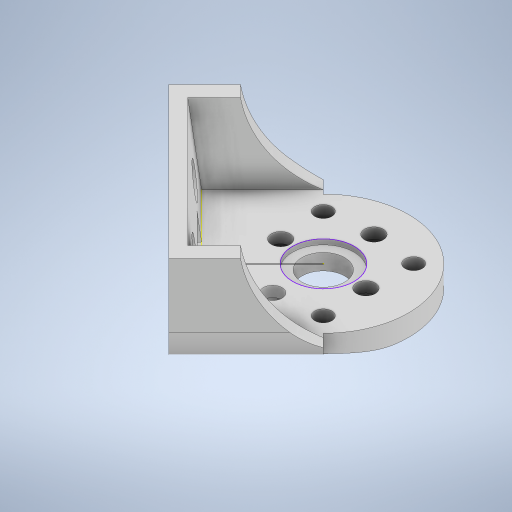
# Autodesk Inventor part: SoporteV4
Saved by Autodesk Inventor 2024 (Build 280153000, 153)
## iProperties
Created: 2023-09-30
Part Number: SoporteV4
Material: Generic
Document SubType Name: Modeling
Designer: felip
Density: 1 g/cm^3
Appearance: Default
Author: felip
Autodesk Inventor part; units mm, degrees
ref_plane "YZ Plane" through (0, 0, 0) normal (1, 0, 0) x (0, 1, 0)
ref_plane "XZ Plane" through (0, 0, 0) normal (0, 1, 0) x (-1, 0, 0)
sketch "Sketch1" plane through (0, 0, 0) normal (0, 1, 0) x (-1, 0, 0)
  line L0 (0, 0) -> (8, 0)
  line L1 (0, 0) -> (-8, 0)
  line L2 (0, 0) -> (0, -9.5)
  line L3 (0, -9.5) -> (0, 9.5)
  circle A0 centre (0, 0) radius 16
  circle A1 centre (0, 9.5) radius 1.75
  circle A2 centre (8, 0) radius 1.75
  circle A3 centre (0, -9.5) radius 1.75
  circle A4 centre (-8, 0) radius 1.75
  circle A5 centre (0, 0) radius 4
  circle A6 centre (0, -9.5) radius 3
  circle A7 centre (8, 0) radius 3
  circle A8 centre (0, 9.5) radius 3
  circle A9 centre (-8, 0) radius 3
  point P0 (16, 0)
  point P1 (0, 16)
  dimension "d0" = 8
  dimension "d1" = 8
  dimension "d2" = 9.5
  dimension "d3" = 19
  dimension "d4" = 32
  dimension "d5" = 3.5
  dimension "d6" = 3.5
  dimension "d7" = 3.5
  dimension "d8" = 3.5
  dimension "d9" = 8
  dimension "d10" = 6
  dimension "d11" = 6
  dimension "d12" = 6
  dimension "d13" = 6
  constraints: 10 centre point, 10 coincident, 8 end point, 2 horizontal, 2 point on circle, 1 point on line, 1 vertical
  measures "d0" distance of L0.start L0.end
  measures "d1" distance of L0.start L1.end
  measures "d2" distance of L0.start L2.end
  measures "d3" distance of L2.end L3.end
  measures "d4" diameter of A0
  measures "d5" diameter of A1
  measures "d6" diameter of A2
  measures "d7" diameter of A3
  measures "d8" diameter of A4
  measures "d9" diameter of A5
  measures "d10" diameter of A6
  measures "d11" diameter of A7
  measures "d12" diameter of A8
  measures "d13" diameter of A9
extrude "Extrusion1" add sketch "Sketch1" along normal blind 4 contours A0
sketch "Sketch3" plane through (0, 4, 0) normal (0, 1, 0) x (1, 0, 0)
  circle A0 centre (0, -9.5) radius 3 projected
  circle A1 centre (0, -9.5) radius 1.75
  circle A2 centre (-8, 0) radius 3 projected
  circle A3 centre (-8, 0) radius 1.75
  circle A4 centre (0, 9.5) radius 3 projected
  circle A5 centre (0, 9.5) radius 1.75
  circle A6 centre (8, 0) radius 3 projected
  circle A7 centre (8, 0) radius 1.75
  point P0 (0, 0)
  dimension "d16" = 3.5
  dimension "d17" = 3.5
  dimension "d18" = 3.5
  dimension "d19" = 3.5
  constraints: 4 centre point, 4 coincident
  measures "d16" diameter of A1
  measures "d17" diameter of A3
  measures "d18" diameter of A5
  measures "d19" diameter of A7
extrude "Extrusion2" add sketch "Sketch3" against normal blind 2
sketch "Sketch5" plane through (0, 0, 0) normal (0, -1, 0) x (1, 0, 0)
  line L0 (0, 0) -> (-4, 0)
  circle A0 centre (0, 0) radius 4 projected
  line L1 (0, 0) -> (0, 4)
  line L2 (0, 0) -> (-14.8492, 14.8492)
  line L3 (0, 0) -> (21, 0) construction
  line L4 (-14.8492, 14.8492) -> (-21.9203, 7.7782)
  line L5 (-14.8492, 14.8492) -> (-7.7782, 21.9203)
  line L6 (-21.9203, 7.7782) -> (-15.683, 1.5408)
  line L7 (-7.7782, 21.9203) -> (-0.7071, 14.8492)
  line L8 (-0.7071, 14.8492) -> (-15.683, 1.5408)
  point P0 (-8.195, 8.195)
  point P1 (-2.8284, 2.8284)
  dimension "d22" = 21
  dimension "d23" = 135
  dimension "d24" = 10
  dimension "d28" = 10
  constraints: 18 end point, 2 horizontal, 2 point on circle, 1 equal length, 1 vertical
  measures "d22" distance of L1.start L2.end
  measures "d23" angle of L3 L2
  measures "d24" distance of L2.end L4.end
  measures "d28" distance of L2.end L5.end
extrude "Extrusion3" add sketch "Sketch5" against normal blind 5 contours L8 L6 L4 L2 | L2 L5 L7 L8
sketch "Sketch6" plane through (0, 0, 0) normal (0, -1, 0) x (1, 0, 0)
  line L0 (-21.9203, 7.7782) -> (-7.7782, 21.9203) projected
  line L1 (-7.7782, 21.9203) -> (-21.9203, 7.7782)
  line L2 (-21.9203, 7.7782) -> (-19.799, 5.6569)
  line L3 (-19.799, 5.6569) -> (-5.6569, 19.799)
  line L4 (-5.6569, 19.799) -> (-7.7782, 21.9203)
  point P0 (0, 0)
  dimension "d31" = 20
  dimension "d32" = 3
  constraints: 8 end point, 2 parallel, 1 perpendicular, 1 point on line
  measures "d31" distance of L0.end L1.end
  measures "d32" distance of L2.end L1.end
extrude "Extrusion4" add sketch "Sketch6" along normal blind 17
sketch "Sketch7" plane through (0, 0, 0) normal (0, -1, 0) x (1, 0, 0)
  circle A0 centre (0, 0) radius 4 projected
  line L0 (0, 0) -> (-10.6066, 10.6066)
  line L1 (0, 0) -> (15, 0) construction
  dimension "d36" = 15
  dimension "d37" = 135
  constraints: 4 end point, 1 equal length, 1 horizontal
  measures "d36" distance of L0.start L0.end
  measures "d37" angle of L1 L0
sketch "Sketch8" plane through (-5.6569, -17, 19.799) normal (0.7071068, 0, -0.7071068) x (-0.7071068, 0, -0.7071068)
  line L0 (10, 17) -> (10, 0)
  line L1 (20, 0) -> (0, 0) projected
  constraints: 2 end point, 1 midpoint
ref_plane "Work Plane3" through (0, 0, 0) normal (0.7071068, 0, 0.7071068) x (-0.7071068, 0, 0.7071068)
sketch "Sketch11" plane through (-5.6569, -17, 19.799) normal (0.7071068, 0, -0.7071068) x (-0.7071068, 0, -0.7071068)
  line L0 (0, 17) -> (20, 17) projected
  line L1 (20, 22) -> (20, 0) projected
  line L2 (0, 17) -> (20, 17)
  line L3 (20, 17) -> (20, 2)
  line L4 (20, 2) -> (0, 2)
  line L5 (0, 2) -> (0, 17)
  line L6 (0, 17) -> (4, 17)
  line L7 (4, 17) -> (4, 14)
  line L8 (4, 14) -> (4, 6)
  line L9 (4, 6) -> (16, 6)
  line L10 (16, 6) -> (16, 14)
  circle A0 centre (4, 14) radius 1.75
  circle A1 centre (4, 6) radius 1.75
  circle A2 centre (16, 6) radius 1.75
  circle A3 centre (16, 14) radius 1.75
  point P0 (10, 17)
  point P1 (8.5, 15)
  dimension "d48" = 4
  dimension "d49" = 3
  dimension "d50" = 8
  dimension "d51" = 12
  dimension "d52" = 8
  dimension "d53" = 3.5
  dimension "d54" = 3.5
  dimension "d55" = 3.5
  dimension "d56" = 3.5
  constraints: 18 end point, 4 centre point, 4 coincident, 3 perpendicular, 2 horizontal, 2 parallel, 2 point on line, 1 vertical, 1 other
  measures "d48" distance of L2.start L6.end
  measures "d49" distance of L6.end L7.end
  measures "d50" distance of L7.end L8.end
  measures "d51" distance of L8.end L9.end
  measures "d52" distance of L9.end L10.end
  measures "d53" diameter of A0
  measures "d54" diameter of A1
  measures "d55" diameter of A2
  measures "d56" diameter of A3
extrude "Extrusion7" cut sketch "Sketch11" against normal blind 5 contours A0 L8 L7 | L7 L8 A0 | A1 L9 L8 | L8 L9 A1 | A2 L10 L9 | L9 L10 A2 | A3
sketch "Sketch12" plane through (0, 0, 0) normal (0, -1, 0) x (1, 0, 0)
  line L0 (0, 0) -> (-8.4853, -8.4853)
  line L1 (0, 0) -> (12, 0) construction
  circle A0 centre (-8.4853, -8.4853) radius 1.6
  line L2 (0, 0) -> (8.4853, -8.4853)
  circle A1 centre (8.4853, -8.4853) radius 1.6
  line L3 (0, 0) -> (8.4853, 8.4853)
  circle A2 centre (8.4853, 8.4853) radius 1.6
  line L4 (0, 0) -> (-8.4853, 8.4853)
  circle A3 centre (-8.4853, 8.4853) radius 1.6
  line L5 (0, 0) -> (-11.5258, 11.5258)
  line L6 (0, 0) -> (11.5258, 11.5258)
  line L7 (11.5258, 11.5258) -> (-11.5258, 11.5258)
  dimension "d60" = 12
  dimension "d61" = 135
  dimension "d62" = 3.2
  dimension "d63" = 12
  dimension "d64" = 3.2
  dimension "d65" = 12
  dimension "d66" = 3.2
  dimension "d69" = 12
  dimension "d70" = 3.2
  dimension "d71" = 16.3
  dimension "d75" = 16.3
  constraints: 16 end point, 4 centre point, 4 coincident, 2 horizontal, 2 point on line, 1 equal length
  measures "d60" distance of L0.start L0.end
  measures "d61" angle of L0 L1
  measures "d62" diameter of A0
  measures "d63" distance of L0.start L2.end
  measures "d64" diameter of A1
  measures "d65" distance of L3.start L3.end
  measures "d66" diameter of A2
  measures "d69" distance of L3.start L4.end
  measures "d70" diameter of A3
  measures "d71" distance of L3.start L5.end
  measures "d75" distance of L3.start L6.end
sketch "Sketch13" plane through (0, 4, 0) normal (0, 1, 0) x (1, 0, 0)
  circle A0 centre (0, 0) radius 5.75
  dimension "d72" = 11.5
  constraints: 1 centre point, 1 coincident
  measures "d72" diameter of A0
extrude "Extrusion8" cut sketch "Sketch13" against normal blind 1
sketch "Sketch14" plane through (-1.7398, 0, 15.882) normal (0.7071068, 0, 0.7071068) x (0.7071068, 0, -0.7071068)
  line L0 (-8.5395, 5) -> (-8.5395, -17) projected
  line L1 (-8.5395, -17) -> (-8.5395, 5)
  line L2 (-8.5395, 5) -> (6.4605, 5)
  line L3 (3.6299, 5) -> (-0.0177, 5) projected
  line L4 (6.4605, 5) -> (-8.5395, -17)
  point P0 (12.4605, 0)
  dimension "d76" = 15
  constraints: 6 end point, 1 collinear, 1 point on line
  measures "d76" distance of L0.start L2.end
extrude "Extrusion9" add sketch "Sketch14" along normal blind 3
fillet "Fillet3" radius 1 3 edges at (-5.6569, -14.8, 19.799) (-6.7175, -17, 20.8597) (-1.53, -8.4401, 19.9147)
sketch "Sketch15" plane through (-15.683, 0, 1.5408) normal (-0.7071068, 0, -0.7071068) x (-0.7071068, 0, 0.7071068)
  line L0 (8.821, 5) -> (8.821, -17) projected
  line L1 (8.821, -17) -> (8.821, 5)
  line L2 (8.821, 5) -> (-6.179, 5)
  line L3 (-6.179, 5) -> (8.821, -17)
  point P0 (-12.179, 0)
  dimension "d80" = 15
  constraints: 6 end point, 1 perpendicular, 1 vertical
  measures "d80" distance of L0.start L2.end
extrude "Extrusion10" add sketch "Sketch15" along normal blind 3
fillet "Fillet4" radius 1 3 edges at (-19.799, -14.8, 5.6569) (-20.8597, -17, 6.7175) (-19.9147, -8.4401, 1.53)
extrude "Extrusion11" cut sketch "Sketch12" against normal blind 6 contours A0 | A1 | A2 L6 L3 | L3 L6 A2 | A3 L5 L4 | L4 L5 A3
sketch "Sketch16" plane through (0, 5, 0) normal (0, 1, 0) x (1, 0, 0)
  line L0 (-5.6569, -24.0416) -> (-24.0416, -5.6569) projected
  line L1 (-24.0416, -5.6569) -> (-13.3457, 5.0391)
  line L2 (-13.3457, 5.0391) -> (5.0391, -13.3457)
  line L3 (5.0391, -13.3457) -> (-5.6569, -24.0416)
  line L4 (-5.6569, -24.0416) -> (-24.0416, -5.6569)
  point P0 (0, 0)
  point P1 (-5.6569, -24.0416)
  constraints: 8 end point, 2 parallel, 2 perpendicular
extrude "Extrusion12" cut sketch "Sketch16" against normal blind 1
sketch "Sketch17" plane through (0, 4, 0) normal (0, 1, 0) x (1, 0, 0)
  line L0 (-17.21, -2.4586) -> (-13.6377, 2.2484)
  line L1 (-13.6377, 2.2484) -> (-11.5469, 0.6617)
  line L2 (-11.5469, 0.6617) -> (-15.1192, -4.0453)
  line L3 (-15.1192, -4.0453) -> (-17.21, -2.4586)
  point P0 (0, 0)
  constraints: 8 end point, 2 parallel, 1 perpendicular
extrude "Extrusion13" add sketch "Sketch17" against normal blind 4
sketch "Sketch18" plane through (-5.6569, -12.6, 19.799) normal (0.7071068, 0, -0.7071068) x (-0.7071068, 0, -0.7071068)
  line L0 (10, 12.6) -> (10, -4.4)
  line L1 (19, -4.4) -> (1, -4.4) projected
  line L2 (10, 12.6) -> (10, 4.1)
  line L3 (10, 4.1) -> (24.9533, 4.1)
  line L4 (24.9533, 4.1) -> (-2.995, 4.1)
  line L5 (24.9533, 4.1) -> (-3.5693, 4.1)
  line L6 (-3.5693, 4.1) -> (-3.5693, -4.8148)
  line L7 (-3.5693, -4.8148) -> (24.9533, -4.8148)
  line L8 (24.9533, -4.8148) -> (24.9533, 4.1)
  point P0 (10, 4.1)
  dimension "d90" = 8.5
  constraints: 16 end point, 2 midpoint, 2 parallel, 2 perpendicular, 1 horizontal, 1 point on line
  measures "d90" distance of L0.start L2.end
extrude "Extrusion14" cut sketch "Sketch18" along normal mid plane 10
fillet "Fillet5" radius 2 1 edges at (-12.7279, -8.5, 12.7279)
sketch "Sketch19" plane through (0, 0, 0) normal (0, -1, 0) x (1, 0, 0)
  line L0 (0, 0) -> (12.0208, 12.0208)
  line L1 (0, 0) -> (17, 0) construction
  line L2 (0, 0) -> (-12.0208, -12.0208)
  line L3 (0, 0) -> (-14.8492, 14.8492)
  line L4 (-5.6569, 24.0416) -> (-24.0416, 5.6569) projected
  line L5 (-14.8492, 14.8492) -> (-26.8701, 2.8284)
  line L6 (-26.8701, 2.8284) -> (-12.0208, -12.0208)
  line L7 (-14.8492, 14.8492) -> (-2.8284, 26.8701)
  line L8 (-2.8284, 26.8701) -> (12.0208, 12.0208)
  arc A0 (-15.8638, -2.0835) -> (2.0835, 15.8638) centre (0, 0) ccw projected
  line L9 (-23.8901, 5.8084) -> (-13.0815, -5.0003)
  line L10 (-13.0815, -5.0003) -> (-11.3137, -11.3137)
  line L11 (-6.0104, 23.6881) -> (6.62, 11.0576)
  line L12 (6.62, 11.0576) -> (11.3137, 11.3137)
  point P0 (-15.8425, -2.2392)
  point P1 (-24.0416, 5.6569)
  dimension "d96" = 17
  dimension "d97" = 45
  dimension "d98" = 17
  dimension "d99" = 17
  dimension "d100" = 17
  constraints: 24 end point, 6 point on line, 3 perpendicular, 2 point on circle, 1 equal length, 1 horizontal, 1 midpoint
  measures "d96" distance of L0.start L0.end
  measures "d97" angle of L1 L0
  measures "d98" distance of L0.start L2.end
  measures "d99" distance of L3.end L5.end
  measures "d100" distance of L3.end L7.end
extrude "Extrusion15" add sketch "Sketch19" against normal blind 4 contours L12 L11 L4 L7 L8 L0 | L2 L6 L5 L4 L9 A0
sketch "Sketch21" plane through (0, 0, 0) normal (0, -1, 0) x (1, 0, 0)
  line L0 (12.0208, 12.0208) -> (-2.8284, 26.8701) projected
  line L1 (12.0208, 12.0208) -> (14.1421, 14.1421)
  line L2 (12.0208, 12.0208) -> (15.0208, 12.0208) construction
  line L3 (14.1421, 14.1421) -> (-0.7071, 28.9914)
  line L4 (-0.7071, 28.9914) -> (-2.8284, 26.8701)
  line L5 (-2.8284, 26.8701) -> (-5.6569, 24.0416) projected
  line L6 (-2.8284, 26.8701) -> (12.0208, 12.0208)
  line L7 (-11.3137, -11.3137) -> (-12.0208, -12.0208) projected
  line L8 (-12.0208, -12.0208) -> (-14.1421, -14.1421)
  line L9 (-14.1421, -14.1421) -> (-28.9914, 0.7071)
  line L10 (-26.8701, 2.8284) -> (-12.0208, -12.0208) projected
  line L11 (-28.9914, 0.7071) -> (-26.8701, 2.8284)
  line L12 (-26.8701, 2.8284) -> (-12.0208, -12.0208)
  line L13 (-0.7071, 28.9914) -> (1.4142, 26.8701)
  line L14 (1.4142, 26.8701) -> (-26.8701, -1.4142)
  line L15 (-28.9914, 0.7071) -> (-0.7071, 28.9914)
  point P0 (0, 0)
  point P1 (-24.7487, 0.7071)
  point P2 (-0.7071, 24.7487)
  dimension "d109" = 3
  dimension "d110" = 45
  dimension "d111" = 3
  dimension "d112" = 21
  dimension "d113" = 3
  constraints: 24 end point, 5 perpendicular, 2 collinear, 2 point on line, 1 equal length, 1 horizontal
  measures "d109" distance of L0.start L1.end
  measures "d110" angle of L2 L1
  measures "d111" distance of L7.end L8.end
  measures "d112" distance of L8.end L9.end
  measures "d113" distance of L3.end L13.end
extrude "Extrusion16" add sketch "Sketch21" against normal blind 19
draft "FaceDraft1" angle 7 pull direction (0, 1, 0) faces at (-16.7349, 9, 8.721) fixed edges at (-12.7279, 19, 12.7279)
sketch "Sketch22" plane through (-28.9914, 0, 0.7071) normal (-0.7071068, 0, -0.7071068) x (-0.7071068, 0, 0.7071068)
  line L0 (0, 0) -> (0, 19) projected
  line L1 (0, 19) -> (-10, 19)
  line L2 (0, 19) -> (-21, 19) projected
  line L3 (-4.8418, 4) -> (-21, 4) projected
  arc A0 (-21, 4) -> (-10, 19) centre (-29.7782, 21.9706) ccw
  line L4 (-21, 0) -> (-21, 19) projected
  line L5 (-21, 4) -> (-21, 19)
  line L6 (-21, 19) -> (-10, 19)
  dimension "d117" = 10
  dimension "d118" = 20
  constraints: 6 end point, 2 point on circle, 1 centre point, 1 collinear, 1 perpendicular, 1 point on line
  measures "d117" distance of L0.end L1.end
  measures "d118" radius of A0
extrude "Extrusion17" cut sketch "Sketch22" against normal blind 50
sketch "Sketch23" plane through (0.5952, 4, 23.4464) normal (0.7018361, 0.1218693, -0.7018361) x (-0.7071068, 0, -0.7071068)
  line L0 (17, 0.0546) -> (17, 15.1126)
  line L1 (0, 15.1126) -> (34, 15.1126) projected
  line L2 (17, 0.0546) -> (17, 7.5546)
  line L3 (17, 7.5546) -> (8.5, 7.5546)
  line L4 (17, 7.5546) -> (25.5, 7.5546)
  circle A0 centre (25.5, 7.5546) radius 1.75
  circle A1 centre (8.5, 7.5546) radius 1.75
  point P0 (17, -5.9394)
  dimension "d122" = 7.5
  dimension "d123" = 8.5
  dimension "d124" = 8.5
  dimension "d125" = 3.5
  dimension "d126" = 3.5
  constraints: 8 end point, 2 centre point, 2 coincident, 1 horizontal, 1 midpoint, 1 perpendicular, 1 point on line
  measures "d122" distance of L0.start L2.end
  measures "d123" distance of L2.end L3.end
  measures "d124" distance of L2.end L4.end
  measures "d125" diameter of A0
  measures "d126" diameter of A1
extrude "Extrusion18" cut sketch "Sketch23" against normal blind 10
sketch "Sketch24" plane through (0.5952, 4, 23.4464) normal (0.7018361, 0.1218693, -0.7018361) x (-0.7071068, 0, -0.7071068)
  circle A0 centre (25.5, 7.5546) radius 1.75 projected
  circle A1 centre (25.5, 7.5546) radius 3
  circle A2 centre (8.5, 7.5546) radius 1.75 projected
  circle A3 centre (8.5, 7.5546) radius 3
  point P0 (17, -5.9394)
  dimension "d129" = 6
  dimension "d130" = 6
  constraints: 2 centre point, 2 coincident
  measures "d129" diameter of A1
  measures "d130" diameter of A3
extrude "Extrusion19" cut sketch "Sketch24" against normal blind 1 contours A0 | A1 | A2 | A3
sketch "Sketch25" plane through (-24.0416, -8.5, 5.6569) normal (-0.7071068, 0, 0.7071068) x (0.7071068, 0, 0.7071068)
  line L0 (36.138, -0.923) -> (-10.7057, -0.923)
  line L1 (-10.7057, -0.923) -> (-10.7057, 30.1299)
  line L2 (-10.7057, 30.1299) -> (36.138, 30.1299)
  line L3 (36.138, 30.1299) -> (36.138, -0.923)
  point P0 (13, 8.5)
  constraints: 8 end point, 2 parallel, 1 horizontal, 1 perpendicular
extrude "Extrusion20" cut sketch "Sketch25" against normal blind 0.5
sketch "Sketch26" plane through (-19.2365, -8.5, 2.266) normal (0, -1, 0) x (0.7071068, 0, -0.7071068)
  point P0 (15.2045, 12)
sketch "Sketch27" plane through (-19.2365, -8.5, 2.266) normal (0, -1, 0) x (0.7071068, 0, -0.7071068)
  line L0 (-9.8497, 36.5928) -> (35.4602, 36.5928)
  line L1 (35.4602, 36.5928) -> (35.4602, -13.7002)
  line L2 (35.4602, -13.7002) -> (-9.8497, -13.7002)
  line L3 (-9.8497, -13.7002) -> (-9.8497, 36.5928)
  point P0 (15.2045, 12)
  constraints: 8 end point, 2 parallel, 1 horizontal, 1 perpendicular
extrude "Extrusion21" cut sketch "Sketch27" against normal blind 8.5
fillet "Fillet8" radius 7 2 edges at (-21.3893, 0, -6.895) (6.895, 0, 21.3893)
sketch "Sketch28" plane through (0.5952, 4, 23.4464) normal (0.7018361, 0.1218693, -0.7018361) x (-0.7071068, 0, -0.7071068)
  point P0 (17, -5.9394)
sketch "Sketch29" plane through (0, 4, 0) normal (0, 1, 0) x (1, 0, 0)
  circle A0 centre (0, 0) radius 5.75
  line L0 (0, 0) -> (-11.4256, -11.4256)
  line L1 (-23.4464, 0.5952) -> (0.5952, -23.4464) projected
  constraints: 2 end point, 1 centre point, 1 coincident, 1 midpoint
sketch "Sketch30" plane through (0.5952, 4, 23.4464) normal (0.7018361, 0.1218693, -0.7018361) x (-0.7071068, 0, -0.7071068)
  line L0 (34, 0) -> (0, 0) projected
  line L1 (17, 0) -> (22, 0)
  line L2 (17, 0) -> (12, 0)
  line L3 (12, 0) -> (12, 5)
  line L4 (12, 5) -> (22, 5)
  line L5 (22, 5) -> (22, 0)
  point P0 (17, -5.9394)
  dimension "d139" = 5
  dimension "d140" = 5
  dimension "d141" = 5
  constraints: 10 end point, 3 perpendicular, 2 point on line, 1 midpoint
  measures "d139" distance of L1.start L1.end
  measures "d140" distance of L1.start L2.end
  measures "d141" distance of L2.end L3.end
extrude "Extrusion22" cut sketch "Sketch30" against normal blind 10
body "Solid1"
